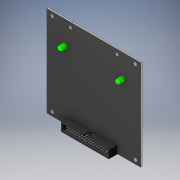
# Autodesk Inventor part: Rev Board
Saved by Autodesk Inventor 2017 (Build 210142000, 142)
## iProperties
Created: 2016-12-13
Part Number: Rev Board
Material: Generic
Document SubType Name: Modeling
Designer: Roksbot
Density: 1 g/cm^3
Appearance: Default
Author: Roksbot
Autodesk Inventor part; units mm, degrees
ref_plane "YZ Plane" through (0, 0, 0) normal (1, 0, 0) x (0, 1, 0)
ref_plane "XZ Plane" through (0, 0, 0) normal (0, 1, 0) x (-1, 0, 0)
ref_plane "XY Plane" through (0, 0, 0) normal (0, 0, 1) x (1, 0, 0)
sketch "Sketch1" plane through (0, 0, 0) normal (0, 0, 1) x (1, 0, 0)
  line L0 (49.9872, -48.2981) -> (-49.9872, -48.2981)
  line L1 (-49.9872, -48.2981) -> (-49.9872, 48.2981)
  line L2 (-49.9872, 48.2981) -> (49.9872, 48.2981)
  line L3 (49.9872, 48.2981) -> (49.9872, -48.2981)
  line L4 (49.9872, -48.2981) -> (-49.9872, 48.2981) construction
  line L5 (-49.9872, -48.2981) -> (49.9872, 48.2981) construction
  line L6 (0, 48.2981) -> (0, -48.2981) construction
  circle A0 centre (-44.2722, 44.2595) radius 1.905
  circle A1 centre (-24.8412, 43.2181) radius 1.778
  circle A2 centre (-44.2722, -44.2595) radius 1.905
  circle A3 centre (44.2722, 44.2595) radius 1.905
  circle A4 centre (24.8412, 43.2181) radius 1.778
  circle A5 centre (44.2722, -44.2595) radius 1.905
  point P0 (0, 0)
  dimension "d0" = 96.5962
  dimension "d1" = 99.9744
  dimension "d2" = 2.1336
  dimension "d3" = 3.81
  dimension "d4" = 2.1336
  dimension "d5" = 3.81
  dimension "d6" = 3.556
  dimension "d7" = 3.302
  dimension "d8" = 23.368
  constraints: 14 end point, 6 centre point, 4 midpoint, 3 symmetric about line, 2 parallel, 1 equal radius, 1 horizontal, 1 perpendicular, 1 vertical alignment, 3 other
  measures "d0" distance of L0.end L1.end
  measures "d1" distance of L1.end L2.end
  measures "d2" distance edge to line of A0 L2
  measures "d3" distance edge to line of A0 L1
  measures "d4" distance edge to line of A2 L0
  measures "d5" diameter of A2
  measures "d6" diameter of A1
  measures "d7" distance edge to line of A1 L2
  measures "d8" distance edge to line of A1 L1
extrude "Extrusion1" add sketch "Sketch1" along normal blind 1.4224
sketch "Sketch2" plane through (0, 0, 1.4224) normal (0, 0, 1) x (1, 0, 0)
  circle A0 centre (-30.6578, 23.5839) radius 2.8194
  circle A1 centre (30.6578, 23.5839) radius 2.8194
  line L0 (-49.9872, 48.2981) -> (49.9872, 48.2981) construction
  line L1 (0, 48.2981) -> (0, 0) construction
  line L2 (-49.9872, 48.2981) -> (-49.9872, -48.2981) construction
  dimension "d11" = 5.6388
  dimension "d12" = 27.5336
  dimension "d13" = 16.51
  constraints: 2 centre point, 2 end point, 1 horizontal alignment, 1 midpoint, 1 vertical, 1 other
  measures "d11" diameter of A0
  measures "d13" distance edge to line of A0 L2
extrude "Extrusion2" add sketch "Sketch2" along normal blind 0.762
sketch "Sketch3" plane through (-30.6578, 23.5839, 2.1844) normal (0, 0, 1) x (1, 0, 0)
  circle A0 centre (0, 0) radius 2.8194 projected
  circle A1 centre (61.3156, 0) radius 2.8194 projected
  circle A2 centre (0, 0) radius 2.5019
  circle A3 centre (61.3156, 0) radius 2.5019
  point P0 (30.6578, -23.5839)
  dimension "d16" = 5.0038
  constraints: 2 centre point, 2 coincident, 1 equal radius
  measures "d16" diameter of A2
extrude "Extrusion3" add sketch "Sketch3" along normal blind 6.0452 contours A2 | A3
fillet "Fillet1" radius 2.5019 2 edges at (-33.1597, 23.5839, 8.2296) (28.1559, 23.5839, 8.2296)
sketch "Sketch4" plane through (0, 0, 1.4224) normal (0, 0, 1) x (1, 0, 0)
  line L0 (25.4, -48.2727) -> (-25.4, -48.2727)
  line L1 (-25.4, -48.2727) -> (-25.4, -39.6367)
  line L2 (-25.4, -39.6367) -> (25.4, -39.6367)
  line L3 (25.4, -39.6367) -> (25.4, -48.2727)
  line L4 (25.4, -48.2727) -> (-25.4, -39.6367) construction
  line L5 (-25.4, -48.2727) -> (25.4, -39.6367) construction
  line L6 (-49.9872, -48.2981) -> (49.9872, -48.2981) projected
  point P0 (0, 0)
  point P1 (0, -43.9547)
  point P2 (0, -43.9547)
  dimension "d20" = 8.636
  dimension "d21" = 50.8
  dimension "d22" = 0.0254
  constraints: 12 end point, 3 midpoint, 2 parallel, 1 horizontal, 1 perpendicular, 1 vertical alignment
  measures "d20" distance of L2.end L0.start
  measures "d21" distance of L1.end L2.end
  measures "d22" distance between parallel lines of L0 L6
extrude "Extrusion4" add sketch "Sketch4" along normal blind 9.398
sketch "Sketch5" plane through (0, 0, 10.8204) normal (0, 0, 1) x (1, 0, 0)
  line L0 (-25.4, -48.2727) -> (25.4, -48.2727) projected
  line L1 (25.4, -48.2727) -> (25.4, -39.6367) projected
  line L2 (25.4, -39.6367) -> (-25.4, -39.6367) projected
  line L3 (-25.4, -39.6367) -> (-25.4, -48.2727) projected
  line L4 (-24.384, -40.6527) -> (24.384, -40.6527)
  line L5 (24.384, -40.6527) -> (24.384, -47.2567)
  line L6 (24.384, -47.2567) -> (-24.384, -47.2567)
  line L7 (-24.384, -47.2567) -> (-24.384, -40.6527)
  line L8 (2.286, -39.6367) -> (-2.286, -39.6367)
  line L9 (-2.286, -39.6367) -> (-2.286, -40.6527)
  line L10 (-2.286, -40.6527) -> (2.286, -40.6527)
  line L11 (2.286, -40.6527) -> (2.286, -39.6367)
  line L12 (2.286, -39.6367) -> (-2.286, -40.6527) construction
  line L13 (-2.286, -39.6367) -> (2.286, -40.6527) construction
  point P0 (0, 0)
  point P1 (0, -40.1447)
  point P2 (0, -40.1447)
  dimension "d25" = 1.016
  dimension "d26" = 4.572
  constraints: 20 end point, 3 midpoint, 2 parallel, 2 point on line, 1 horizontal, 1 perpendicular, 1 vertical alignment, 3 other
  measures "d25" distance between parallel lines of L2 L4
  measures "d26" distance from line of L8.start L9
extrude "Extrusion5" cut sketch "Sketch5" against normal blind 6.7564 contours L2 L11 L4 L9 | L4 L5 L6 L7
chamfer "Chamfer1" distance 0.508 angle 45 5 edges at (-13.335, -40.6527, 10.8204) (-24.384, -43.9547, 10.8204) (0, -47.2567, 10.8204) (24.384, -43.9547, 10.8204) (13.335, -40.6527, 10.8204)
sketch "Sketch6" plane through (0, 0, 4.064) normal (0, 0, 1) x (1, 0, 0)
  line L0 (-20.6375, -42.3672) -> (-20.0025, -42.3672)
  line L1 (-20.0025, -42.3672) -> (-20.0025, -43.0022)
  line L2 (-20.0025, -43.0022) -> (-20.6375, -43.0022)
  line L3 (-20.6375, -43.0022) -> (-20.6375, -42.3672)
  line L4 (-20.6375, -42.3672) -> (-20.0025, -43.0022) construction
  line L5 (-20.0025, -42.3672) -> (-20.6375, -43.0022) construction
  line L6 (-24.384, -47.2567) -> (-24.384, -40.6527) projected
  line L7 (-24.384, -43.9547) -> (24.384, -43.9547) construction
  line L8 (24.384, -40.6527) -> (24.384, -47.2567) projected
  line L9 (24.384, -47.2567) -> (-24.384, -47.2567) projected
  line L10 (0, -47.2567) -> (0, -39.6367) construction
  line L11 (-2.286, -39.6367) -> (2.286, -39.6367) projected
  point P0 (0, 0)
  point P1 (-20.32, -42.6847)
  dimension "d32" = 0.635
  dimension "d34" = 1.27
  dimension "d35" = 20.32
  constraints: 16 end point, 6 midpoint, 2 parallel, 2 perpendicular, 1 horizontal
  measures "d32" distance of L0.start L0.end
  measures "d34" distance from line of L7 point (-20.32, -42.685)
  measures "d35" distance from line of L10 point (-20.32, -42.685)
extrude "Extrusion6" add sketch "Sketch6" along normal blind 6.4262
chamfer "Chamfer2" distance 0.254 angle 45 4 edges at (-20.32, -43.0022, 10.4902) (-20.0025, -42.6847, 10.4902) (-20.32, -42.3672, 10.4902) (-20.6375, -42.6847, 10.4902)
pattern_linear "Rectangular Pattern1" count 17 spacing 2.54 along (1, 0, 0) count 2 spacing 2.54 along (0, -1, 0) of "Extrusion6", "Chamfer2"
equation "\"d4\" = d2"
body "Solid1"
